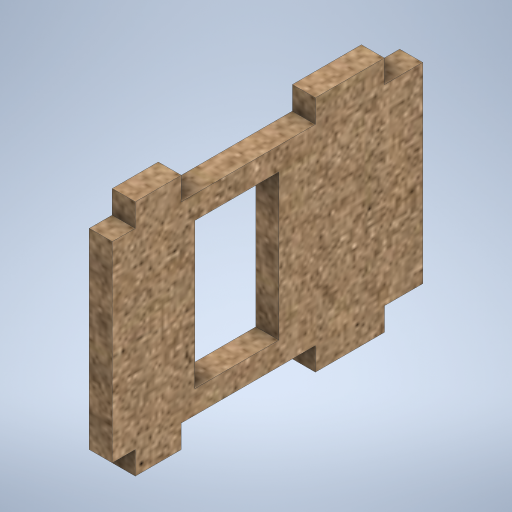
# Autodesk Inventor part: Switch_Support
Saved by Autodesk Inventor 2024 (Build 280153000, 153)
## iProperties
Created: 2023-11-23
Part Number: Switch_Support
Material: MDF Tablero de fibras de densidad media
Document SubType Name: Modeling
Designer: marco
Density: 0.8 g/cm^3
Appearance: Cartón - Ondulado
Author: marco
Autodesk Inventor part; units mm, degrees
ref_plane "YZ Plane" through (0, 0, 0) normal (1, 0, 0) x (0, 1, 0)
ref_plane "XZ Plane" through (0, 0, 0) normal (0, 1, 0) x (-1, 0, 0)
ref_plane "XY Plane" through (0, 0, 0) normal (0, 0, 1) x (1, 0, 0)
sketch "Boceto1" plane through (0, 0, 0) normal (1, 0, 0) x (0, 1, 0)
  line L0 (12.5, 11.25) -> (12.5, 8)
  line L1 (12.5, -6.25) -> (12.5, 11.25)
  line L2 (-12.5, 11.25) -> (-12.5, -6.25)
  line L3 (-15.5, -9.25) -> (-15.5, -6.25)
  line L4 (12.5, 11.25) -> (15.5, 11.25)
  line L5 (15.5, 11.25) -> (15.5, 17.25)
  line L6 (-15.5, 17.25) -> (-15.5, 11.25)
  line L7 (-15.5, 11.25) -> (-12.5, 11.25)
  line L8 (-12.5, 11.25) -> (-12.5, -6.25)
  line L9 (12.5, 11.25) -> (12.5, -6.25)
  line L10 (12.5, -6.25) -> (15.5, -6.25)
  line L11 (15.5, -6.25) -> (15.5, -15.25)
  line L12 (15.5, -15.25) -> (12.5, -15.25)
  line L13 (12.5, -15.25) -> (12.5, -20.25)
  line L14 (12.5, -20.25) -> (-12.5, -20.25)
  line L15 (-12.5, -20.25) -> (-12.5, -15.25)
  line L16 (-12.5, -15.25) -> (-15.5, -15.25)
  line L17 (-15.5, -15.25) -> (-15.5, -6.25)
  line L18 (9.5, 9.5) -> (-9.5, 9.5)
  line L19 (-9.5, 9.5) -> (-9.5, -1.5)
  line L20 (-9.5, -1.5) -> (9.5, -1.5)
  line L21 (9.5, -1.5) -> (9.5, 9.5)
  line L22 (-15.5, -6.25) -> (-15.5, -15.25)
  line L23 (-15.5, -15.25) -> (-12.5, -15.25)
  line L24 (-12.5, -15.25) -> (-12.5, -20.25)
  line L25 (-12.5, -20.25) -> (12.5, -20.25)
  line L26 (12.5, -20.25) -> (12.5, -15.25)
  line L27 (12.5, -15.25) -> (15.5, -15.25)
  line L28 (15.5, -15.25) -> (15.5, -6.25)
  line L29 (15.5, -6.25) -> (12.5, -6.25)
  line L30 (12.5, -6.25) -> (12.5, 11.25)
  line L31 (12.5, 11.25) -> (15.5, 11.25)
  line L32 (15.5, 11.25) -> (15.5, 17.25)
  line L33 (-15.5, 17.25) -> (-15.5, 11.25)
  line L34 (-15.5, 11.25) -> (-12.5, 11.25)
  line L35 (-12.5, 11.25) -> (-12.5, -6.25)
  line L36 (-12.5, -6.25) -> (-15.5, -6.25)
  line L37 (12.5, 17.25) -> (12.5, 20.25)
  line L38 (12.5, 20.25) -> (-12.5, 20.25)
  line L39 (-12.5, 20.25) -> (-12.5, 17.25)
  line L40 (15.5, 17.25) -> (12.5, 17.25)
  line L41 (-12.5, 17.25) -> (-15.5, 17.25)
  line L42 (15.5, 17.25) -> (12.5, 17.25)
  line L43 (-12.5, 17.25) -> (-15.5, 17.25)
  point P0 (0, 0)
  constraints: 88 end point, 5 perpendicular
extrude "Extrusión1" add sketch "Boceto1" along normal blind 3
